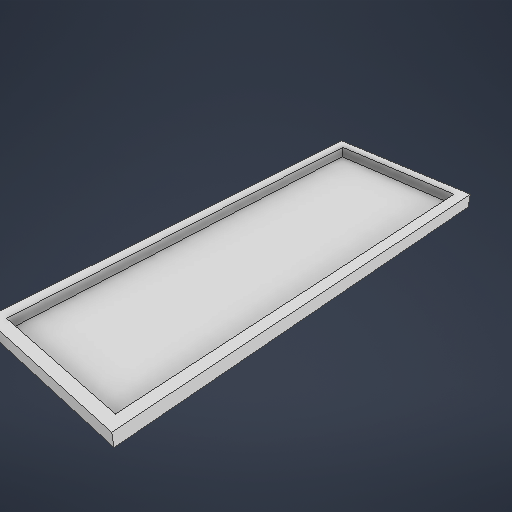
# Autodesk Inventor part: Keyboard-bottom
Saved by Autodesk Inventor 2026.1 (Build 301233000, 233)
## iProperties
Created: 2025-12-14
Part Number: Keyboard-bottom
Material: Generic
Document SubType Name: Modeling
Designer: chest
Density: 1 g/cm^3
Appearance: Default
Author: chest
Autodesk Inventor part; units mm, degrees
ref_plane "YZ Plane" through (0, 0, 0) normal (1, 0, 0) x (0, 1, 0)
ref_plane "XZ Plane" through (0, 0, 0) normal (0, 1, 0) x (-1, 0, 0)
ref_plane "XY Plane" through (0, 0, 0) normal (0, 0, 1) x (1, 0, 0)
sketch "Sketch1" plane through (0, 0, 0) normal (0, 1, 0) x (-1, 0, 0)
  point P0 (0, 0)
sketch "Sketch2" plane through (0, 0, 0) normal (0, 1, 0) x (-1, 0, 0)
  line L0 (0, 0) -> (-144.19, 0)
  line L1 (-144.19, 0) -> (-144.19, -379.14)
  line L2 (-144.19, -379.14) -> (0, -379.14)
  line L3 (0, -379.14) -> (0, 0)
  line L4 (0, 0) -> (-124.19, 0)
  line L5 (-124.19, 0) -> (-124.19, -359.14)
  line L6 (-124.19, -359.14) -> (0, -359.14)
  line L7 (0, -359.14) -> (0, 0)
  dimension "d0" = 144.19
  dimension "d1" = 379.14
  dimension "d2" = 124.19
  dimension "d3" = 359.14
  constraints: 16 end point, 4 parallel, 2 horizontal, 2 perpendicular
  measures "d0" distance of L2.end L1.end
  measures "d1" distance of L1.end L0.end
  measures "d2" distance of L6.end L5.end
  measures "d3" distance of L5.end L4.end
extrude "Extrusion1" add sketch "Sketch2" along normal blind 13
sketch "Sketch3" plane through (0, 13, 0) normal (0, 1, 0) x (1, 0, 0)
  line L0 (10, 10) -> (134.19, 10)
  line L1 (134.19, 10) -> (134.19, 369.14)
  line L2 (134.19, 369.14) -> (10, 369.14)
  line L3 (10, 369.14) -> (10, 10)
  line L4 (144.19, 379.14) -> (0, 379.14) projected
  line L5 (0, 379.14) -> (0, 0) projected
  dimension "d6" = 124.19
  dimension "d7" = 359.14
  dimension "d8" = 10
  dimension "d9" = 10
  constraints: 8 end point, 2 parallel, 1 horizontal, 1 perpendicular
  measures "d6" distance of L2.end L1.end
  measures "d7" distance of L1.end L0.end
  measures "d8" distance between parallel lines of L4 L2
  measures "d9" distance between parallel lines of L5 L3
extrude "Extrusion2" cut sketch "Sketch3" against normal blind 10
body "Solid1"
